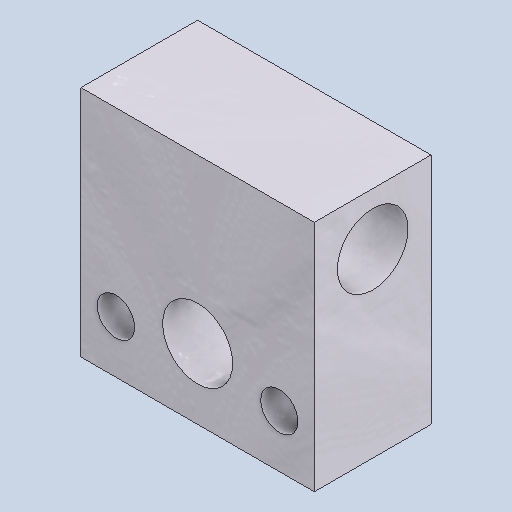
# Autodesk Inventor part: ENDER 3 HEATBLOCK
Saved by Autodesk Inventor 2022 (Build 260153070, 153G)
## iProperties
Created: 2022-01-01
Part Number: ENDER 3 HEATBLOCK
Material: Aluminum 6061, Welded
Document SubType Name: Modeling
Designer: a laptop
Density: 2.7 g/cm^3
Appearance: Weld - Aluminum
Author: a laptop
Autodesk Inventor part; units mm, degrees
ref_plane "YZ Plane" through (0, 0, 0) normal (1, 0, 0) x (0, 1, 0)
ref_plane "XZ Plane" through (0, 0, 0) normal (0, 1, 0) x (-1, 0, 0)
ref_plane "XY Plane" through (0, 0, 0) normal (0, 0, 1) x (1, 0, 0)
sketch "Sketch1" plane through (0, 0, 0) normal (0, 0, 1) x (1, 0, 0)
  line L0 (-10, 10) -> (10, 10)
  line L1 (10, 10) -> (10, -10)
  line L2 (10, -10) -> (-10, -10)
  line L3 (-10, -10) -> (-10, 10)
  point P0 (0, 0)
  dimension "d0" = 20
  dimension "d1" = 10
  dimension "d2" = 10
  dimension "d3" = 10
  constraints: 8 end point, 2 parallel, 1 horizontal, 1 perpendicular
  measures "d0" distance of L0.start L0.end
  measures "d1" distance from line of L1 point (0, 0)
  measures "d2" distance from line of point (0, 0) L0
  measures "d3" distance from line of point (0, 0) L2
extrude "Extrusion1" add sketch "Sketch1" along normal blind 10
sketch "Sketch2" plane through (0, 0, 0) normal (0, 0, -1) x (-1, 0, 0)
  circle A0 centre (0, -4) radius 3
  line L0 (0, -4) -> (0, 0) construction
  circle A1 centre (-7, -5.5) radius 1.6
  circle A2 centre (7, -5.5) radius 1.6
  dimension "d6" = 6
  dimension "d7" = 4
  dimension "d8" = 3.2
  dimension "d9" = 7
  dimension "d10" = 5.5
  constraints: 3 centre point, 2 end point, 1 symmetric about line, 1 vertical, 1 vertical alignment, 1 other
  measures "d6" diameter of A0
  measures "d7" distance of L0.start L0.end
  measures "d8" diameter of A1
  measures "d9" distance from line of L0 A1.centre
  measures "d10" vertical distance of L0.end A1.centre
sketch "Sketch3" plane through (10, -10, 0) normal (1, 0, 0) x (0, 0, -1)
  circle A0 centre (-5, 15.5) radius 3.025
  point P0 (0, 10)
  point P1 (0, 0)
  dimension "d11" = 6.05
  dimension "d12" = 5
  dimension "d13" = 15.5
  constraints: 1 centre point
  measures "d11" diameter of A0
  measures "d12" horizontal distance of point (0, 0) A0.centre
  measures "d13" vertical distance of point (0, 0) A0.centre
extrude "Extrusion2" cut sketch "Sketch3" against normal blind 20
extrude "Extrusion3" cut sketch "Sketch2" against normal blind 10
body "Solid1"
